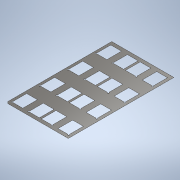
# Autodesk Inventor part: Assembly Stencil
Saved by Autodesk Inventor 2022 (Build 260153000, 153)
## iProperties
Created: 2021-01-11
Part Number: Assembly Stencil
Material: Stainless Steel
Document SubType Name: Modeling
Designer: caleb
Density: 8 g/cm^3
Appearance: Semi-Polished
Author: caleb
Autodesk Inventor part; units mm, degrees
ref_plane "YZ Plane" through (0, 0, 0) normal (1, 0, 0) x (0, 1, 0)
ref_plane "XZ Plane" through (0, 0, 0) normal (0, 1, 0) x (-1, 0, 0)
ref_plane "XY Plane" through (0, 0, 0) normal (0, 0, 1) x (1, 0, 0)
sketch "Sketch1" plane through (0, 0, 0) normal (0, 1, 0) x (-1, 0, 0)
  line L0 (-63.5, 107.95) -> (63.5, 107.95)
  line L1 (63.5, 107.95) -> (63.5, -107.95)
  line L2 (63.5, -107.95) -> (-63.5, -107.95)
  line L3 (-63.5, -107.95) -> (-63.5, 107.95)
  line L4 (-63.5, 107.95) -> (63.5, -107.95) construction
  line L5 (63.5, 107.95) -> (-63.5, -107.95) construction
  point P0 (0, 0)
  dimension "d0" = 215.9
  dimension "d1" = 127
  constraints: 12 end point, 2 midpoint, 2 parallel, 1 horizontal, 1 perpendicular
  measures "d0" distance of L0.end L1.end
  measures "d1" distance of L0.start L0.end
extrude "Extrusion1" add sketch "Sketch1" along normal blind 0.1
chamfer "Chamfer1" distance 3.175 angle 45 1 edges at (-63.5, 0.05, 107.95)
sketch "Sketch2" plane through (0, 0.1, 0) normal (0, 1, 0) x (1, 0, 0)
  line L0 (-36.5, -100.95) -> (-36.5, -70.95)
  line L1 (-36.5, -70.95) -> (-58.5, -70.95)
  line L2 (-63.5, 107.95) -> (-63.5, -107.95) projected
  line L3 (-63.5, -107.95) -> (63.5, -107.95) projected
  arc A0 (-58.5, -99.45) -> (-57, -100.95) centre (-58.5, -100.95) ccw
  line L4 (-36.5, -100.95) -> (-57, -100.95)
  line L5 (-58.5, -99.45) -> (-58.5, -70.95)
  line L6 (57.5, -70.95) -> (35.5, -70.95)
  line L7 (35.5, -70.95) -> (35.5, -100.95)
  arc A1 (56, -100.95) -> (57.5, -99.45) centre (57.5, -100.95) ccw
  line L8 (57.5, -70.95) -> (57.5, -99.45)
  line L9 (63.5, -107.95) -> (63.5, 107.95) projected
  line L10 (35.5, -100.95) -> (56, -100.95)
  line L11 (-36.5, -43.633) -> (-36.5, -13.633)
  line L12 (-36.5, -43.633) -> (-57, -43.633)
  line L13 (-36.5, -13.633) -> (-58.5, -13.633)
  line L14 (-58.5, -42.133) -> (-58.5, -13.633)
  arc A2 (-58.5, -42.133) -> (-57, -43.633) centre (-58.5, -43.633) ccw
  line L15 (-36.5, 13.684) -> (-36.5, 43.684)
  line L16 (-36.5, 13.684) -> (-57, 13.684)
  line L17 (-36.5, 43.684) -> (-58.5, 43.684)
  line L18 (-58.5, 15.184) -> (-58.5, 43.684)
  arc A3 (-58.5, 15.184) -> (-57, 13.684) centre (-58.5, 13.684) ccw
  line L19 (-36.5, 71.001) -> (-36.5, 101.001)
  line L20 (-36.5, 71.001) -> (-57, 71.001)
  line L21 (-36.5, 101.001) -> (-58.5, 101.001)
  line L22 (-58.5, 72.501) -> (-58.5, 101.001)
  arc A4 (-58.5, 72.501) -> (-57, 71.001) centre (-58.5, 71.001) ccw
  line L23 (-2.5, -100.95) -> (-2.5, -70.95)
  line L24 (-2.5, -100.95) -> (-23, -100.95)
  line L25 (-2.5, -70.95) -> (-24.5, -70.95)
  line L26 (-24.5, -99.45) -> (-24.5, -70.95)
  arc A5 (-24.5, -99.45) -> (-23, -100.95) centre (-24.5, -100.95) ccw
  line L27 (-2.5, -43.633) -> (-2.5, -13.633)
  line L28 (-2.5, -43.633) -> (-23, -43.633)
  line L29 (-2.5, -13.633) -> (-24.5, -13.633)
  line L30 (-24.5, -42.133) -> (-24.5, -13.633)
  arc A6 (-24.5, -42.133) -> (-23, -43.633) centre (-24.5, -43.633) ccw
  line L31 (-2.5, 13.684) -> (-2.5, 43.684)
  line L32 (-2.5, 13.684) -> (-23, 13.684)
  line L33 (-2.5, 43.684) -> (-24.5, 43.684)
  line L34 (-24.5, 15.184) -> (-24.5, 43.684)
  arc A7 (-24.5, 15.184) -> (-23, 13.684) centre (-24.5, 13.684) ccw
  line L35 (-2.5, 71.001) -> (-2.5, 101.001)
  line L36 (-2.5, 71.001) -> (-23, 71.001)
  line L37 (-2.5, 101.001) -> (-24.5, 101.001)
  line L38 (-24.5, 72.501) -> (-24.5, 101.001)
  arc A8 (-24.5, 72.501) -> (-23, 71.001) centre (-24.5, 71.001) ccw
  arc A9 (56, -43.633) -> (57.5, -42.133) centre (57.5, -43.633) ccw
  line L39 (57.5, -13.633) -> (35.5, -13.633)
  line L40 (35.5, -13.633) -> (35.5, -43.633)
  line L41 (57.5, -13.633) -> (57.5, -42.133)
  line L42 (35.5, -43.633) -> (56, -43.633)
  arc A10 (56, 13.684) -> (57.5, 15.184) centre (57.5, 13.684) ccw
  line L43 (57.5, 43.684) -> (35.5, 43.684)
  line L44 (35.5, 43.684) -> (35.5, 13.684)
  line L45 (57.5, 43.684) -> (57.5, 15.184)
  line L46 (35.5, 13.684) -> (56, 13.684)
  arc A11 (56, 71.001) -> (57.5, 72.501) centre (57.5, 71.001) ccw
  line L47 (57.5, 101.001) -> (35.5, 101.001)
  line L48 (35.5, 101.001) -> (35.5, 71.001)
  line L49 (57.5, 101.001) -> (57.5, 72.501)
  line L50 (35.5, 71.001) -> (56, 71.001)
  arc A12 (22, -100.95) -> (23.5, -99.45) centre (23.5, -100.95) ccw
  line L51 (23.5, -70.95) -> (1.5, -70.95)
  line L52 (1.5, -70.95) -> (1.5, -100.95)
  line L53 (23.5, -70.95) -> (23.5, -99.45)
  line L54 (1.5, -100.95) -> (22, -100.95)
  arc A13 (22, -43.633) -> (23.5, -42.133) centre (23.5, -43.633) ccw
  line L55 (23.5, -13.633) -> (1.5, -13.633)
  line L56 (1.5, -13.633) -> (1.5, -43.633)
  line L57 (23.5, -13.633) -> (23.5, -42.133)
  line L58 (1.5, -43.633) -> (22, -43.633)
  arc A14 (22, 13.684) -> (23.5, 15.184) centre (23.5, 13.684) ccw
  line L59 (23.5, 43.684) -> (1.5, 43.684)
  line L60 (1.5, 43.684) -> (1.5, 13.684)
  line L61 (23.5, 43.684) -> (23.5, 15.184)
  line L62 (1.5, 13.684) -> (22, 13.684)
  arc A15 (22, 71.001) -> (23.5, 72.501) centre (23.5, 71.001) ccw
  line L63 (23.5, 101.001) -> (1.5, 101.001)
  line L64 (1.5, 101.001) -> (1.5, 71.001)
  line L65 (23.5, 101.001) -> (23.5, 72.501)
  line L66 (1.5, 71.001) -> (22, 71.001)
  dimension "d46" = 1.5
  dimension "d47" = 30
  dimension "d50" = 7
  dimension "d51" = 5
  dimension "d54" = 30
  dimension "d55" = 30
  dimension "d56" = 6
  dimension "d58" = 1.5
  dimension "d59" = 7
  dimension "d62" = 57.317
  dimension "d65" = 34
  dimension "d70" = 57.317
  dimension "d73" = 34
  dimension "d77" = 22
  dimension "d78" = 22
  constraints: 128 end point, 32 point on circle, 16 centre point, 4 collinear, 4 horizontal, 4 vertical, 2 horizontal alignment, 2 perpendicular, 1 parallel, 1 vertical alignment, 150 other
  measures "d46" radius of A0
  measures "d47" distance of L1.end A0.centre
  measures "d50" distance between parallel lines of L3 L4
  measures "d51" distance between parallel lines of L2 L5
  measures "d54" distance of L6.start A1.centre
  measures "d55" distance of L6.end L7.end
  measures "d56" distance between parallel lines of L9 L8
  measures "d58" radius of A1
  measures "d59" distance between parallel lines of L3 L10
  measures "d62" distance of L0.end L11.end
  measures "d65" distance of L0.end L23.end
  measures "d70" distance of L10.end L42.end
  measures "d73" distance of L10.end L54.end
  measures "d77" distance between parallel lines of L0 L5
  measures "d78" distance between parallel lines of L7 L8
extrude "Extrusion2" cut sketch "Sketch2" against normal through all
equation "\"d54\" = d47"
equation "\"d55\" = d47"
equation "\"d59\" = d50"
equation "\"d73\" = d65"
equation "\"d78\" = d77"
body "Solid1"
